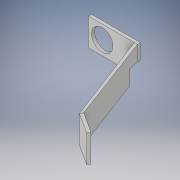
# Autodesk Inventor part: Spinner to Top Other Side
Saved by Autodesk Inventor 2017 (Build 210142000, 142)
## iProperties
Created: 2017-06-10
Part Number: Spinner to Top Other Side
Material: Generic
Document SubType Name: Modeling
Designer: Matthew
Density: 1 g/cm^3
Appearance: Default
Author: Matthew
Autodesk Inventor part; units mm, degrees
ref_plane "YZ Plane" through (0, 0, 0) normal (1, 0, 0) x (0, 1, 0)
ref_plane "XZ Plane" through (0, 0, 0) normal (0, 1, 0) x (-1, 0, 0)
sketch "Sketch1" plane through (0, 0, 0) normal (0, 1, 0) x (-1, 0, 0)
  line L0 (43.0137, 64.3915) -> (32.1817, 14.8739)
  line L1 (-10.5502, -12.5966) -> (-8.8333, -15.2673)
  line L2 (-8.8333, -15.2673) -> (35.0028, 12.913)
  line L3 (35.0028, 12.913) -> (46.1153, 63.713)
  line L4 (46.1153, 63.713) -> (43.0137, 64.3915)
  line L5 (-10.5502, -12.5966) -> (-10.5502, 12.913)
  line L6 (-10.5502, -12.5966) -> (32.1817, 14.8739)
  line L7 (46.1153, 63.713) -> (74.6903, 63.713)
  line L8 (74.6903, 63.713) -> (74.6903, 66.888)
  line L9 (74.6903, 66.888) -> (43.5598, 66.888)
  line L10 (43.0137, 64.3915) -> (43.5598, 66.888)
  point P0 (0, 0)
  dimension "d0" = 3.175
  dimension "d1" = 3.175
  dimension "d3" = 50.8
  dimension "d4" = 57.265
  dimension "d5" = 50.8
  dimension "d6" = 11.1125
  dimension "d7" = 28.575
  dimension "d8" = 3.175
  constraints: 22 end point, 4 perpendicular, 3 vertical, 1 collinear, 1 horizontal, 1 parallel, 1 other
  measures "d0" distance of L1.start L1.end
  measures "d1" distance of L3.end L0.start
  measures "d3" distance of L1.start L0.end
  measures "d4" angle of L5 L6
  measures "d5" vertical distance of L2.end L3.end
  measures "d6" horizontal distance of L2.end L3.end
  measures "d7" distance of L3.end L7.end
  measures "d8" distance of L7.end L8.end
extrude "Extrusion1" add sketch "Sketch1" along normal blind 28.575
sketch "Sketch2" plane through (-74.6903, 0, 66.888) normal (0, 0, 1) x (1, 0, 0)
  line L0 (28.575, 0) -> (0, 0) projected
  line L1 (0, 0) -> (0, 28.575) projected
  line L2 (28.575, 28.575) -> (0, 28.575) projected
  line L3 (28.575, 0) -> (28.575, 28.575) projected
  line L4 (28.575, 28.575) -> (0, 28.575) projected
  line L5 (0, 0) -> (0, 28.575) projected
  circle A0 centre (14.2875, 14.2875) radius 11.1125
  point P0 (74.6903, 0)
  point P1 (14.2875, 28.575)
  point P2 (0, 14.2875)
  dimension "d11" = 22.225
  constraints: 2 midpoint, 1 centre point
  measures "d11" diameter of A0
extrude "Extrusion2" cut sketch "Sketch2" against normal blind 28.575 contours A0
sketch "Sketch3" plane through (10.5502, 0, -12.5966) normal (0.5407576, 0, 0.8411785) x (0.8411785, 0, -0.5407576)
  line L0 (-50.8, 0) -> (-50.8, 28.575) projected
  line L1 (-50.8, 7.9375) -> (0, 7.9375)
  line L2 (0, 7.9375) -> (0, -20.6375)
  line L3 (0, -20.6375) -> (-50.8, -20.6375)
  line L4 (-50.8, -20.6375) -> (-50.8, 7.9375)
  line L5 (-50.8, 28.575) -> (0, 28.575) projected
  point P0 (-15.6863, 0)
  dimension "d14" = 50.8
  dimension "d15" = 28.575
  dimension "d16" = 20.6375
  constraints: 8 end point, 2 parallel, 1 horizontal, 1 perpendicular, 1 point on line
  measures "d14" distance of L2.end L3.end
  measures "d15" distance of L1.end L2.end
  measures "d16" distance from line of L5 L1.end
sketch "Sketch4" plane through (-32.1817, 0, 14.8739) normal (0.9769, 0, 0.2136969) x (0.2136969, 0, -0.9769)
  line L0 (-53.2441, 0) -> (-53.2441, 28.575) projected
  line L1 (-53.2441, 28.575) -> (0, 7.9375)
  line L2 (0, 0) -> (0, 28.575) projected
  line L3 (0, 7.9375) -> (0, -20.6375)
  line L4 (0, -20.6375) -> (-53.2441, 0)
  line L5 (-53.2441, 28.575) -> (-53.2441, 0)
  point P0 (21.4074, 0)
  dimension "d17" = 20.6375
  dimension "d18" = 28.575
  constraints: 8 end point, 1 collinear, 1 point on line, 1 vertical
  measures "d17" distance of L2.end L1.end
  measures "d18" distance of L1.end L3.end
sketch "Sketch5" plane through (-32.1817, 0, 14.8739) normal (0.9769, 0, 0.2136969) x (0.2136969, 0, -0.9769)
  line L0 (-53.2441, 41.9678) -> (42.8737, 41.9678)
  line L1 (42.8737, 41.9678) -> (42.8737, -28.4609)
  line L2 (42.8737, -28.4609) -> (-53.2441, -28.4609)
  line L3 (-53.2441, -28.4609) -> (-53.2441, 41.9678)
  point P0 (21.4074, 0)
  constraints: 8 end point, 2 parallel, 1 horizontal, 1 perpendicular
extrude "Extrusion3" cut sketch "Sketch5" along normal blind 50.8 and the other way blind 3.175
extrude "Extrusion4" add sketch "Sketch4" against normal blind 3.175
extrude "Extrusion5" add sketch "Sketch3" against normal blind 3.175
sketch "Sketch6" plane through (8.8333, 0, -15.2673) normal (-0.5407576, 0, -0.8411785) x (-0.8411785, 0, 0.5407576)
  line L0 (50.8, 7.9375) -> (0, 7.9375) projected
  line L1 (50.8, 7.9375) -> (63.8738, 7.9375)
  line L2 (63.8738, 7.9375) -> (63.8738, -20.6375)
  line L3 (63.8738, -20.6375) -> (50.8, -20.6375)
  line L4 (50.8, -20.6375) -> (50.8, 7.9375)
  point P0 (15.6863, 0)
  constraints: 8 end point, 2 parallel, 1 horizontal, 1 perpendicular
extrude "Extrusion6" add sketch "Sketch6" against normal blind 3.175
sketch "Sketch7" plane through (-35.2833, 0, 14.1954) normal (-0.9769, 0, -0.2136969) x (-0.2136969, 0, 0.9769)
  line L0 (50.6885, 27.5845) -> (0, 7.9375) projected
  line L1 (3.1832, -19.4037) -> (53.2441, 0) projected
  line L2 (0, 7.9375) -> (3.1832, 7.9375) projected
  line L3 (0, 7.9375) -> (-56.9759, -14.1465)
  line L4 (-56.9759, -14.1465) -> (-50.1301, -40.068)
  line L5 (53.2441, 0) -> (0, -20.6375) projected
  line L6 (-50.1301, -40.068) -> (0, -20.6375)
  line L7 (0, 7.9375) -> (-35.9676, 7.9375) projected
  line L8 (0, 7.9375) -> (0, -20.6375)
  line L9 (11.5155, 12.4009) -> (21.1446, -12.4418)
  line L10 (-34.1585, 31.8696) -> (27.6424, 31.8696)
  line L11 (27.6424, 31.8696) -> (27.6424, -37.0154)
  line L12 (27.6424, -37.0154) -> (-34.1585, -37.0154)
  line L13 (-34.1585, -37.0154) -> (-34.1585, 31.8696)
  point P0 (-21.4074, 0)
  constraints: 18 end point, 3 perpendicular, 2 collinear, 2 parallel, 2 point on line, 1 horizontal
extrude "Extrusion7" cut sketch "Sketch7" along normal blind 25.4 contours L9 L1 L5 L8 L0 | L0 L7 L13 L10 L11 | L0 L11 L1 L9 | L8 L6 L13 L3 | L3 L13 L7 | L1 L11 L12 L13 L6 L5
mirror "Mirror1" about plane through (-74.6903, 0, 66.888) normal (0, 0, 1)
sketch "Sketch8" plane through (0, 28.575, 0) normal (0, 1, 0) x (1, 0, 0)
  line L0 (-74.6903, -63.713) -> (-74.6903, -70.063) projected
  line L1 (-74.6903, -66.888) -> (15.7413, -66.888)
  line L2 (15.7413, -66.888) -> (15.7413, 23.0839)
  line L3 (15.7413, 23.0839) -> (-74.6903, 23.0839)
  line L4 (-74.6903, 23.0839) -> (-74.6903, -66.888)
  point P0 (0, 0)
  constraints: 8 end point, 2 parallel, 1 horizontal, 1 midpoint, 1 perpendicular
extrude "Extrusion8" cut sketch "Sketch8" against normal blind 49.2125
ref_plane "Work Plane1" through (-7.3684, -20.6375, 113.4742) normal (0.9769, 0, -0.2136969) x (-0.2136969, 0, -0.9769)
sketch "Sketch10" plane through (0, 28.575, 0) normal (0, 1, 0) x (1, 0, 0)
  line L0 (-1.9264, -138.3519) -> (-5.0281, -139.0304)
  line L1 (-1.9264, -138.3519) -> (-13.3045, -86.3378) projected
  line L2 (-46.6614, -54.5282) -> (-5.0281, -54.5282)
  line L3 (-5.0281, -54.5282) -> (-5.0281, -144.0467)
  line L4 (-5.0281, -144.0467) -> (-46.6614, -144.0467)
  line L5 (-46.6614, -144.0467) -> (-46.6614, -54.5282)
  point P0 (0, 0)
  dimension "d35" = 3.175
  constraints: 10 end point, 2 parallel, 2 perpendicular, 1 horizontal
  measures "d35" distance of L0.start L0.end
extrude "Extrusion9" cut sketch "Sketch10" against normal blind 57.15 contours L3 L4 L5 L2
sketch "Sketch11" plane through (0, 28.575, 0) normal (0, 1, 0) x (1, 0, 0)
  line L0 (-74.6903, -66.888) -> (-46.6614, -66.888) projected
  line L1 (-46.6614, -66.888) -> (-46.1153, -66.888)
  line L2 (-46.1153, -66.888) -> (-46.1153, -70.063)
  line L3 (-46.1153, -70.063) -> (-46.6614, -70.063)
  line L4 (-46.6614, -70.063) -> (-46.6614, -66.888)
  line L5 (-74.6903, -66.888) -> (-74.6903, -70.063) projected
  point P0 (0, 0)
  dimension "d38" = 28.575
  constraints: 8 end point, 2 parallel, 1 horizontal, 1 perpendicular
  measures "d38" distance between parallel lines of L5 L2
extrude "Extrusion10" add sketch "Sketch11" against normal up to surface (28.575 mm away)
sketch "Sketch12" plane through (-74.6903, 0, 66.888) normal (0, 0, -1) x (-1, 0, 0)
  line L0 (0, 0) -> (-28.575, 0) projected
  line L1 (0, 28.575) -> (0, 0) projected
  line L2 (-28.575, 28.575) -> (0, 28.575) projected
  line L3 (-28.575, 28.575) -> (-28.575, 0) projected
  circle A0 centre (-14.2875, 14.2875) radius 11.1125 projected
  point P0 (-74.6903, 0)
extrude "Extrusion11" add sketch "Sketch12" along normal blind 6.35
sketch "Sketch13" plane through (-74.6903, 0, 70.063) normal (0, 0, 1) x (1, 0, 0)
  line L0 (28.575, 28.575) -> (0, 28.575) projected
  line L1 (0, 0) -> (0, 28.575) projected
  line L2 (28.575, 0) -> (0, 0) projected
  line L3 (28.575, 28.575) -> (28.575, 0) projected
  circle A0 centre (14.2875, 14.2875) radius 11.1125 projected
  point P0 (74.6903, 0)
extrude "Extrusion12" cut sketch "Sketch13" against normal blind 6.35
sketch "Sketch14" plane through (-7.3684, -20.6375, 113.4742) normal (0.9769, 0, -0.2136969) x (-0.2136969, 0, -0.9769)
  line L0 (-22.8553, 28.575) -> (-26.5426, 28.575) projected
  line L1 (59.9935, 49.2125) -> (59.9935, 20.6375) projected
  line L2 (-22.8553, 28.575) -> (59.9935, 49.2125)
  line L3 (59.9935, 20.6375) -> (66.0999, 20.6375) projected
  line L4 (59.9935, 49.2125) -> (59.9935, 20.6375)
  line L5 (-22.8553, 0) -> (-22.8553, 28.575) projected
  line L6 (59.9935, 20.6375) -> (-22.8553, 0)
  line L7 (-22.8553, 0) -> (-22.8553, 28.575)
  point P0 (109.2784, 20.6375)
  constraints: 8 end point, 2 equal length, 1 perpendicular
extrude "Extrusion13" add sketch "Sketch14" against normal blind 3.175
sketch "Sketch16" plane through (-46.1153, 0, 60.538) normal (1, 0, 0) x (0, 0, -1)
  line L0 (-3.175, 28.575) -> (-3.175, 0) projected
  line L1 (-3.175, 0) -> (0, 0) projected
  line L2 (0, 28.575) -> (0, 0) projected
  line L3 (-3.175, 28.575) -> (0, 28.575) projected
  point P0 (60.538, 0)
extrude "Extrusion14" add sketch "Sketch16" along normal blind 33.3375
sketch "Sketch17" plane through (-7.3684, -20.6375, 113.4742) normal (0.9769, 0, -0.2136969) x (-0.2136969, 0, -0.9769)
  line L0 (39.8727, 61.7245) -> (70.5453, 61.7245)
  line L1 (70.5453, 61.7245) -> (70.5453, 3.8032)
  line L2 (70.5453, 3.8032) -> (39.8727, 3.8032)
  line L3 (39.8727, 3.8032) -> (39.8727, 61.7245)
  point P0 (109.2784, 20.6375)
  constraints: 8 end point, 2 parallel, 1 horizontal, 1 perpendicular
extrude "Extrusion15" cut sketch "Sketch17" along normal blind 33.3375
sketch "Sketch18" plane through (0, 28.575, 0) normal (0, 1, 0) x (1, 0, 0)
  line L0 (-74.6903, -60.538) -> (-18.9482, -60.538) projected
  line L1 (-26.1324, -60.538) -> (-14.0387, -60.538)
  line L2 (-14.0387, -60.538) -> (-14.0387, -48.514)
  line L3 (-14.0387, -48.514) -> (-26.1324, -48.514)
  line L4 (-26.1324, -48.514) -> (-26.1324, -60.538)
  point P0 (0, 0)
  constraints: 8 end point, 2 parallel, 1 horizontal, 1 perpendicular, 1 point on line
extrude "Extrusion16" cut sketch "Sketch18" against normal blind 33.3375
sketch "Sketch19" plane through (0, 28.575, 0) normal (0, 1, 0) x (1, 0, 0)
  line L0 (-21.5038, -63.713) -> (-74.6903, -63.713) projected
  line L1 (-28.5092, -63.713) -> (0.9764, -63.713)
  line L2 (0.9764, -63.713) -> (0.9764, -136.358)
  line L3 (0.9764, -136.358) -> (-28.5092, -136.358)
  line L4 (-28.5092, -136.358) -> (-28.5092, -63.713)
  point P0 (0, 0)
  constraints: 8 end point, 2 parallel, 1 horizontal, 1 perpendicular, 1 point on line
extrude "Extrusion17" cut sketch "Sketch19" against normal blind 82.55
sketch "Sketch20" plane through (0, 28.575, 0) normal (0, 1, 0) x (1, 0, 0)
  line L0 (-74.6903, -60.538) -> (-22.1983, -60.538) projected
  line L1 (-21.5038, -63.713) -> (-74.6903, -63.713) projected
  line L2 (-74.6903, -60.538) -> (-23.8903, -60.538)
  line L3 (-23.8903, -60.538) -> (-23.8903, -63.713)
  line L4 (-23.8903, -63.713) -> (-74.6903, -63.713)
  line L5 (-74.6903, -63.713) -> (-74.6903, -60.538)
  line L6 (-23.8903, -55.4967) -> (-9.2163, -55.4967)
  line L7 (-9.2163, -55.4967) -> (-9.2163, -75.9107)
  line L8 (-9.2163, -75.9107) -> (-23.8903, -75.9107)
  line L9 (-23.8903, -75.9107) -> (-23.8903, -55.4967)
  point P0 (0, 0)
  dimension "d55" = 50.8
  constraints: 16 end point, 4 parallel, 2 horizontal, 2 perpendicular, 1 point on line
  measures "d55" distance of L3.end L4.end
extrude "Extrusion18" cut sketch "Sketch20" against normal blind 82.55 contours L9 L6 L7 L8 L3
sketch "Sketch21" plane through (-5.0281, 7.9375, 140.1325) normal (0, 1, 0) x (1, 0, 0)
  line L0 (15.5783, -6.2401) -> (13.8614, -8.9109) projected
  line L1 (13.8614, -8.9109) -> (15.5783, -6.2401)
  line L2 (15.5783, -6.2401) -> (-5.7877, 7.4951)
  line L3 (-5.7877, 7.4951) -> (-7.5046, 4.8244)
  line L4 (-7.5046, 4.8244) -> (13.8614, -8.9109)
  point P0 (5.0281, 140.1325)
  dimension "d58" = 25.4
  constraints: 8 end point, 3 equal length, 1 perpendicular
  measures "d58" distance of L2.end L0.start
extrude "Extrusion19" add sketch "Sketch21" against normal blind 28.575
sketch "Sketch22" plane through (-5.6127, 7.9375, 136.358) normal (0, 1, 0) x (1, 0, 0)
  line L0 (-48.2657, 34.2615) -> (88.3828, 30.5881)
  line L1 (88.3828, 30.5881) -> (85.9509, -59.8767)
  line L2 (85.9509, -59.8767) -> (-50.6975, -56.2034)
  line L3 (-50.6975, -56.2034) -> (-48.2657, 34.2615)
  point P0 (5.6127, 136.358)
  constraints: 8 end point, 2 parallel, 1 perpendicular
extrude "Extrusion20" cut sketch "Sketch22" along normal blind 28.575
sketch "Sketch23" plane through (-74.6903, 0, 63.713) normal (0, 0, 1) x (1, 0, 0)
  line L0 (0, 28.575) -> (50.8, 28.575) projected
  line L1 (50.8, 0) -> (0, 0) projected
  line L2 (50.8, 28.575) -> (47.625, 28.575)
  line L3 (47.625, 28.575) -> (47.625, 0)
  line L4 (47.625, 0) -> (50.8, 0)
  line L5 (50.8, 0) -> (50.8, 28.575)
  point P0 (74.6903, 0)
  dimension "d63" = 3.175
  constraints: 8 end point, 2 parallel, 1 horizontal, 1 perpendicular, 1 point on line
  measures "d63" distance of L4.end L3.end
loft "Loft1" add profiles "Sketch23" section 2 edges at (-11.6742, 7.9375, 133.9728) (-10.8157, -6.35, 132.6374) (-11.6742, -20.6375, 133.9728) (-12.5326, -6.35, 135.3081)
sketch "Sketch26" plane through (-74.6903, 0, 60.538) normal (0, 0, -1) x (-1, 0, 0)
  line L0 (-50.8, 0) -> (-50.8, 28.575) projected
  ellipse E0 centre (-50.8, 0) end of major axis (-31.75, 0) minor radius 12.7
  point P0 (-74.6903, 0)
  dimension "d71" = 12.7
  dimension "d72" = 19.05
  constraints: 2 other
extrude "Extrusion22" cut sketch "Sketch26" against normal blind 12.7
body "Solid1"
